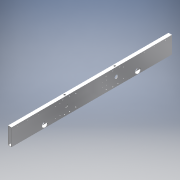
# Autodesk Inventor part: Side Extrusion
Saved by Autodesk Inventor 2019 (Build 230136000, 136)
## iProperties
Created: 2019-10-20
Part Number: Side Extrusion
Material: Aluminum 6061
Document SubType Name: Modeling
Designer: Mark
Density: 2.7 g/cm^3
Appearance: Aluminum - Flat
HoleDistanceX: 199.089 mm
Author: Mark
Autodesk Inventor part; units mm, degrees
ref_plane "YZ Plane" through (0, 0, 0) normal (1, 0, 0) x (0, 1, 0)
ref_plane "XZ Plane" through (0, 0, 0) normal (0, 1, 0) x (-1, 0, 0)
ref_plane "XY Plane" through (0, 0, 0) normal (0, 0, 1) x (1, 0, 0)
sketch "Sketch1" plane through (0, 0, 0) normal (0, 0, 1) x (1, 0, 0)
  line L0 (-10, -50) -> (10, -50)
  line L1 (10, -50) -> (10, 50)
  line L2 (10, 50) -> (-10, 50)
  line L3 (-10, 50) -> (-10, -50)
  line L4 (-10, -50) -> (10, 50) construction
  line L5 (10, -50) -> (-10, 50) construction
  line L6 (-8, -48) -> (8, -48)
  line L7 (8, -48) -> (8, 48)
  line L8 (8, 48) -> (-8, 48)
  line L9 (-8, 48) -> (-8, -48)
  line L10 (-8, -48) -> (8, 48) construction
  line L11 (8, -48) -> (-8, 48) construction
  point P0 (0, 0)
  dimension "d0" = 20
  dimension "d1" = 100
  dimension "d2" = 16
  dimension "d3" = 96
  constraints: 24 end point, 4 midpoint, 4 parallel, 2 horizontal, 2 perpendicular
  measures "d0" distance of L2.end L1.end
  measures "d1" distance of L1.end L0.end
  measures "d2" distance of L8.end L7.end
  measures "d3" distance of L7.end L6.end
extrude "Extrusion1" add sketch "Sketch1" along normal blind 939
sketch "Sketch2" plane through (-10, -50, 0) normal (-1, 0, 0) x (0, 0, 1)
  circle A0 centre (199.089, 18.548) radius 16.3
  line L0 (0, 100) -> (939, 100) projected
  line L1 (0, 100) -> (0, 0) projected
  line L2 (0, 0) -> (939, 0) projected
  point P0 (0, 50)
  dimension "d6" = 32.6
  dimension "HoleDistanceX" = 199.089
  dimension "d11" = 18.548
  constraints: 1 centre point
  measures "d6" diameter of A0
  measures "HoleDistanceX" distance from line of L1 A0.centre
  measures "d11" distance from line of L2 A0.centre
extrude "Extrusion2" cut sketch "Sketch2" against normal blind 880
sketch "Sketch4" plane through (-10, -50, 0) normal (-1, 0, 0) x (0, 0, 1)
  circle A0 centre (113.659, 8.082) radius 4.5 construction
  circle A1 centre (199.089, 18.548) radius 12.25 construction
  line L0 (199.089, 18.548) -> (113.659, 8.082) construction
  line L1 (199.089, 18.548) -> (113.0203, 18.5713) construction
  circle A2 centre (113.0203, 18.5713) radius 4.5 construction
  arc A3 (113.0203, 18.5713) -> (113.659, 8.082) centre (199.089, 18.548) ccw construction
  arc A4 (113.0203, 18.5713) -> (113.659, 8.082) centre (199.089, 18.548) ccw construction
  arc A5 (108.5203, 18.5725) -> (109.1924, 7.5348) centre (199.089, 18.548) ccw
  arc A6 (117.5203, 18.5701) -> (118.1256, 8.6292) centre (199.089, 18.548) ccw
  arc A7 (117.5203, 18.5701) -> (108.5203, 18.5725) centre (113.0203, 18.5713) ccw
  arc A8 (109.1924, 7.5348) -> (118.1256, 8.6292) centre (113.659, 8.082) ccw
  line L2 (0, 0) -> (939, 0) projected
  line L3 (0, 100) -> (0, 0) projected
  point P0 (0, 50)
  dimension "d12" = 9
  dimension "d13" = 9
  dimension "d14" = 9
  dimension "d15" = 7
  dimension "d16" = 8.082
  dimension "d17" = 113.659
  constraints: 12 point on circle, 8 centre point, 4 end point, 4 tangent, 3 coincident, 1 equal length
  measures "d12" diameter of A0
  measures "d13" diameter of A2
  measures "d14" diameter of A7
  measures "d15" angle of L1 L0
  measures "d16" distance from line of L2 L0.end
  measures "d17" distance from line of L3 L0.end
extrude "Extrusion3" cut sketch "Sketch4" against normal blind 3
sketch "Sketch5" plane through (-10, -50, 0) normal (-1, 0, 0) x (0, 0, 1)
  circle A0 centre (325.227, 50) radius 30
  line L0 (0, 100) -> (0, 0) projected
  line L1 (0, 0) -> (939, 0) projected
  point P0 (0, 50)
  dimension "d20" = 60
  dimension "d21" = 325.227
  dimension "d22" = 50
  constraints: 1 centre point
  measures "d20" diameter of A0
  measures "d21" distance from line of L0 A0.centre
  measures "d22" distance from line of L1 A0.centre
extrude "Extrusion4" cut sketch "Sketch5" against normal blind 3
sketch "Sketch6" plane through (-10, -50, 0) normal (-1, 0, 0) x (0, 0, 1)
  line L0 (450, 75) -> (580, 75)
  line L1 (580, 75) -> (580, 25)
  line L2 (580, 25) -> (450, 25)
  line L3 (450, 25) -> (450, 75)
  line L4 (0, 100) -> (939, 100) projected
  line L5 (0, 100) -> (0, 0) projected
  point P0 (0, 50)
  dimension "d25" = 50
  dimension "d26" = 25
  dimension "d27" = 580
  dimension "d28" = 450
  constraints: 8 end point, 2 parallel, 1 horizontal, 1 perpendicular
  measures "d25" distance of L0.end L1.end
  measures "d26" distance between parallel lines of L4 L0
  measures "d27" distance between parallel lines of L5 L1
  measures "d28" distance between parallel lines of L5 L3
extrude "Extrusion5" cut sketch "Sketch6" against normal blind 3
sketch "Sketch7" plane through (8, -48, 0) normal (-1, 0, 0) x (0, 0, 1)
  circle A0 centre (325.227, 48) radius 30 projected
  circle A1 centre (325.227, 48) radius 9.8
  point P0 (0, 48)
  dimension "d31" = 19.6
  constraints: 1 centre point, 1 coincident
  measures "d31" diameter of A1
extrude "Extrusion6" cut sketch "Sketch7" against normal through all contours A1
sketch "Sketch8" plane through (10, -50, 0) normal (1, 0, 0) x (0, 0, -1)
  circle A0 centre (-382.128, 62.7) radius 2.25
  line L0 (0, 100) -> (-939, 100) projected
  line L1 (0, 0) -> (0, 100) projected
  circle A1 centre (-382.128, 37.3) radius 2.25
  line L2 (0, 0) -> (-939, 0) projected
  circle A2 centre (-407.528, 62.7) radius 2.25
  circle A3 centre (-407.528, 37.3) radius 2.25
  point P0 (0, 50)
  dimension "d34" = 4.5
  dimension "d35" = 37.3
  dimension "d36" = 382.128
  dimension "d37" = 4.5
  dimension "d38" = 37.3
  dimension "d39" = 382.128
  dimension "d40" = 4.5
  dimension "d41" = 407.528
  dimension "d42" = 37.3
  dimension "d43" = 4.5
  dimension "d44" = 37.3
  dimension "d45" = 407.528
  constraints: 4 centre point
  measures "d34" diameter of A0
  measures "d35" distance from line of L0 A0.centre
  measures "d36" distance from line of L1 A0.centre
  measures "d37" diameter of A1
  measures "d38" distance from line of L2 A1.centre
  measures "d39" distance from line of L1 A1.centre
  measures "d40" diameter of A2
  measures "d41" distance from line of L1 A2.centre
  measures "d42" distance from line of A2.centre L0
  measures "d43" diameter of A3
  measures "d44" distance from line of L2 A3.centre
  measures "d45" distance from line of L1 A3.centre
extrude "Extrusion7" cut sketch "Sketch8" against normal blind 21.1125
sketch "Sketch9" plane through (10, -50, 0) normal (1, 0, 0) x (0, 0, -1)
  circle A0 centre (-617.924, 50) radius 9.8
  line L0 (0, 100) -> (-939, 100) projected
  line L1 (0, 0) -> (0, 100) projected
  circle A1 centre (-655.408, 80) radius 2.75
  circle A2 centre (-655.408, 20) radius 2.75
  line L2 (0, 0) -> (-939, 0) projected
  circle A3 centre (-562, 84.5) radius 2.75
  circle A4 centre (-562, 15.5) radius 2.75
  circle A5 centre (-283.5, 20) radius 2.75
  circle A6 centre (-283.5, 80) radius 2.75
  circle A7 centre (-384.5, 84.5) radius 2.75
  circle A8 centre (-384.5, 15.5) radius 2.75
  circle A9 centre (-40, 90.5) radius 2.75
  line L3 (-40, 90.5) -> (-160, 90.5)
  line L4 (-40, 90.5) -> (80, 90.5) construction
  circle A10 centre (-160, 90.5) radius 2.75
  circle A11 centre (-100, 90.5) radius 2.75
  circle A12 centre (-903.151, 90.5) radius 2.75
  line L5 (-939, 0) -> (-939, 100) projected
  line L6 (-903.151, 90.5) -> (-843.151, 90.5)
  line L7 (-903.151, 90.5) -> (-843.151, 90.5) construction
  circle A13 centre (-843.151, 90.5) radius 2.75
  line L8 (-843.151, 90.5) -> (-783.151, 90.5)
  line L9 (-843.151, 90.5) -> (-783.151, 90.5) construction
  circle A14 centre (-783.151, 90.5) radius 2.75
  circle A15 centre (-637.924, 90) radius 2.75
  circle A16 centre (-597.924, 90) radius 2.75
  circle A17 centre (-627.924, 10) radius 2.75
  circle A18 centre (-597.924, 10) radius 2.75
  circle A19 centre (-345.226, 90) radius 2.75
  circle A20 centre (-305.226, 90) radius 2.75
  circle A21 centre (-315.226, 10) radius 2.75
  circle A22 centre (-345.226, 10) radius 2.75
  circle A23 centre (-682.408, 80) radius 2.75
  circle A24 centre (-682.408, 20) radius 2.75
  point P0 (0, 50)
  dimension "d48" = 19.6
  dimension "d49" = 50
  dimension "d50" = 617.924
  dimension "d53" = 5.5
  dimension "d54" = 5.5
  dimension "d55" = 20
  dimension "d56" = 20
  dimension "d57" = 655.408
  dimension "d58" = 655.408
  dimension "d60" = 5.5
  dimension "d61" = 5.5
  dimension "d62" = 15.5
  dimension "d63" = 15.5
  dimension "d64" = 562
  dimension "d65" = 562
  dimension "d66" = 5.5
  dimension "d67" = 5.5
  dimension "d68" = 283.5
  dimension "d69" = 283.5
  dimension "d70" = 20
  dimension "d71" = 20
  dimension "d72" = 5.5
  dimension "d73" = 384.5
  dimension "d74" = 15.5
  dimension "d75" = 5.5
  dimension "d76" = 384.5
  dimension "d77" = 15.5
  dimension "d92" = 5.5
  dimension "d93" = 40
  dimension "d94" = 9.5
  dimension "d95" = 120
  dimension "d96" = 180
  dimension "d97" = 5.5
  dimension "d98" = 5.5
  dimension "d99" = 60
  dimension "d100" = 5.5
  dimension "d101" = 35.849
  dimension "d102" = 9.5
  dimension "d103" = 60
  dimension "d104" = 0
  dimension "d105" = 5.5
  dimension "d106" = 60
  dimension "d107" = 0
  dimension "d108" = 5.5
  dimension "d109" = 5.5
  dimension "d110" = 301.076
  dimension "d111" = 10
  dimension "d112" = 5.5
  dimension "d113" = 10
  dimension "d114" = 40
  dimension "d115" = 5.5
  dimension "d116" = 10
  dimension "d117" = 5.5
  dimension "d118" = 10
  dimension "d119" = 40
  dimension "d120" = 30
  dimension "d121" = 5.5
  dimension "d122" = 10
  dimension "d123" = 345.226
  dimension "d124" = 5.5
  dimension "d125" = 40
  dimension "d126" = 10
  dimension "d127" = 5.5
  dimension "d128" = 80
  constraints: 25 centre point, 12 end point, 6 horizontal, 3 coincident, 3 collinear, 1 midpoint
  measures "d48" diameter of A0
  measures "d49" distance from line of L0 A0.centre
  measures "d50" distance from line of L1 A0.centre
  measures "d53" diameter of A1
  measures "d54" diameter of A2
  measures "d55" distance from line of L2 A2.centre
  measures "d56" distance from line of L0 A1.centre
  measures "d57" distance from line of L1 A1.centre
  measures "d58" distance from line of L1 A2.centre
  measures "d60" diameter of A3
  measures "d61" diameter of A4
  measures "d62" distance from line of L2 A4.centre
  measures "d63" distance from line of L0 A3.centre
  measures "d64" distance from line of L1 A3.centre
  measures "d65" distance from line of L1 A4.centre
  measures "d66" diameter of A5
  measures "d67" diameter of A6
  measures "d68" distance from line of L1 A5.centre
  measures "d69" distance from line of L1 A6.centre
  measures "d70" distance from line of L0 A6.centre
  measures "d71" distance from line of L2 A5.centre
  measures "d72" diameter of A7
  measures "d73" distance from line of L1 A7.centre
  measures "d74" distance from line of L0 A7.centre
  measures "d75" diameter of A8
  measures "d76" distance from line of L1 A8.centre
  measures "d77" distance from line of L2 A8.centre
  measures "d92" diameter of A9
  measures "d93" distance from line of L3.start L1
  measures "d94" distance from line of L3.start L0
  measures "d95" distance of L3.start L3.end
  measures "d96" angle of L3 L4
  measures "d97" diameter of A10
  measures "d98" diameter of A11
  measures "d99" distance of A10.centre A11.centre
  measures "d100" diameter of A12
  measures "d101" distance from line of L5 L6.start
  measures "d102" distance from line of L6.start L0
  measures "d103" distance of L6.start L6.end
  measures "d104" distance between parallel lines of L6 L7
  measures "d105" diameter of A13
  measures "d106" distance of L8.start L8.end
  measures "d107" distance between parallel lines of L8 L9
  measures "d108" diameter of A14
  measures "d109" diameter of A15
  measures "d110" distance from line of L5 A15.centre
  measures "d111" distance from line of L0 A15.centre
  measures "d112" diameter of A16
  measures "d113" distance from line of L0 A16.centre
  measures "d114" distance of A15.centre A16.centre
  measures "d115" diameter of A17
  measures "d116" distance from line of L2 A17.centre
  measures "d117" diameter of A18
  measures "d118" distance from line of L2 A18.centre
  measures "d119" horizontal distance of A15.centre A18.centre
  measures "d120" horizontal distance of A17.centre A16.centre
  measures "d121" diameter of A19
  measures "d122" distance from line of L0 A19.centre
  measures "d123" distance from line of L1 A19.centre
  measures "d124" diameter of A20
  measures "d125" distance of A20.centre A19.centre
  measures "d126" distance from line of L0 A20.centre
  measures "d127" diameter of A21
  measures "d128" vertical distance of A20.centre A21.centre
extrude "Extrusion8" cut sketch "Sketch9" against normal blind 37.625 contours A0 | A1 | A2 | A3 | A4 | A5 | A6 | A7 | A8 | A9 | A10 | A11 L3 | L3 A11 | A12 | A14 | A13 L8 L6 | L6 L8 A13 | A15 | A16 | A17 | A18 | A19 | A20 | A21 | A22 | A23 | A24
sketch "Sketch10" plane through (-10, -50, 0) normal (-1, 0, 0) x (0, 0, 1)
  circle A0 centre (744.0619, 18.548) radius 16.3
  line L0 (0, 0) -> (939, 0) projected
  circle A1 centre (199.089, 18.548) radius 16.3 projected
  circle A2 centre (617.924, 50) radius 9.8 projected
  point P0 (0, 50)
  dimension "d78" = 32.6
  dimension "d79" = 18.548
  dimension "d83" = 126.1379
  constraints: 1 centre point
  measures "d78" diameter of A0
  measures "d79" distance from line of L0 A0.centre
  measures "d83" horizontal distance of A2.centre A0.centre
extrude "Extrusion9" cut sketch "Sketch10" against normal through all contours A0
sketch "Sketch11" plane through (-10, 50, 0) normal (0, 1, 0) x (1, 0, 0)
  circle A0 centre (10, -325.227) radius 5
  line L0 (20, 0) -> (0, 0) projected
  line L1 (20, 0) -> (20, -939) projected
  circle A1 centre (10, -617.924) radius 5
  line L2 (20, -939) -> (0, -939) projected
  line L3 (0, 0) -> (0, -939) projected
  point P0 (10, 0)
  dimension "d84" = 10
  dimension "d85" = 325.227
  dimension "d86" = 10
  dimension "d87" = 10
  dimension "d88" = 321.076
  dimension "d89" = 10
  constraints: 2 centre point
  measures "d84" diameter of A0
  measures "d85" distance from line of L0 A0.centre
  measures "d86" distance from line of L1 A0.centre
  measures "d87" diameter of A1
  measures "d88" distance from line of L2 A1.centre
  measures "d89" distance from line of L3 A1.centre
extrude "Extrusion10" cut sketch "Sketch11" against normal blind 10 contours A0 | A1
body "Solid1"
